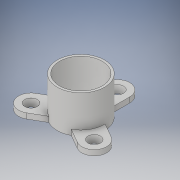
# Autodesk Inventor part: Wood Mount 1 Inch
Saved by Autodesk Inventor 2018 (Build 220112000, 112)
## iProperties
Created: 2018-01-10
Part Number: Wood Mount 1 Inch
Material: Generic
Document SubType Name: Modeling
Designer: owner
Density: 1 g/cm^3
Appearance: Default
Author: owner
Autodesk Inventor part; units mm, degrees
ref_plane "YZ Plane" through (0, 0, 0) normal (1, 0, 0) x (0, 1, 0)
ref_plane "XZ Plane" through (0, 0, 0) normal (0, 1, 0) x (-1, 0, 0)
sketch "Sketch1" plane through (0, 0, 0) normal (0, 1, 0) x (-1, 0, 0)
  circle A0 centre (0, 0) radius 16.7767
  circle A1 centre (0, 0) radius 18.5801
  circle A2 centre (-24.8666, 14.3567) radius 2.413
  circle A3 centre (-24.8666, 14.3567) radius 4.8895
  line L0 (-29.7371, 5.9209) -> (-18.5727, -0.5249)
  line L1 (-19.9962, 22.7926) -> (-8.8318, 16.3469)
  arc A4 (-19.9962, 22.7926) -> (-29.7371, 5.9209) centre (-24.8666, 14.3567) ccw
  circle A5 centre (0, -28.7135) radius 2.413
  circle A6 centre (0, -28.7135) radius 4.8895
  line L2 (-9.7409, -28.7135) -> (-9.7409, -15.822)
  arc A7 (-9.7409, -28.7135) -> (9.7409, -28.7135) centre (0, -28.7135) ccw
  line L3 (9.7409, -28.7135) -> (9.7409, -15.822)
  circle A8 centre (24.8666, 14.3567) radius 2.413
  circle A9 centre (24.8666, 14.3567) radius 4.8895
  line L4 (29.7371, 5.9209) -> (18.5727, -0.5249)
  arc A10 (29.7371, 5.9209) -> (19.9961, 22.7926) centre (24.8666, 14.3567) ccw
  line L5 (19.9961, 22.7926) -> (8.8318, 16.3469)
  point P0 (0, 14.3567)
  point P1 (-16.0908, 9.29)
  constraints: 12 end point, 10 centre point, 7 coincident, 6 point on circle, 1 tangent, 9 other
extrude "Extrusion1" add sketch "Sketch1" along normal blind 29.5402 contours A1
extrude "Extrusion2" add sketch "Sketch1" along normal blind 4.2164 contours A1 L0 A4 L1
extrude "Extrusion3" add sketch "Sketch1" along normal blind 4.2164 contours A1 L5 A10 L4
extrude "Extrusion4" add sketch "Sketch1" along normal blind 4.2164 contours L3 A7 L2 A1
sketch "Sketch2" plane through (0, 4.2164, 0) normal (0, 1, 0) x (1, 0, 0)
  arc A0 (-29.7371, -5.9209) -> (-19.9961, -22.7926) centre (-24.8666, -14.3567) ccw projected
  line L0 (-19.9961, -22.7926) -> (-8.8318, -16.3469) projected
  arc A1 (-18.5727, 0.5249) -> (-8.8318, -16.3469) centre (0, 0) ccw projected
  line L1 (-18.5727, 0.5249) -> (-29.7371, -5.9209) projected
  circle A2 centre (24.8666, -14.3567) radius 4.8895 projected
  circle A3 centre (0, 28.7135) radius 4.8895 projected
  arc A4 (9.7409, 28.7135) -> (-9.7409, 28.7135) centre (0, 28.7135) ccw projected
  line L2 (9.7409, 15.822) -> (9.7409, 28.7135) projected
  line L3 (-9.7409, 28.7135) -> (-9.7409, 15.822) projected
  circle A5 centre (0, 28.7135) radius 2.413 projected
  line L4 (29.7371, -5.9209) -> (18.5727, 0.5249) projected
  arc A6 (19.9962, -22.7926) -> (29.7371, -5.9209) centre (24.8666, -14.3567) ccw projected
  circle A7 centre (24.8666, -14.3567) radius 2.413 projected
  line L5 (8.8318, -16.3469) -> (19.9962, -22.7926) projected
  circle A8 centre (0, 0) radius 18.5801 projected
  circle A9 centre (0, 0) radius 16.7767 projected
ref_plane "Work Plane1" through (-13.7086, 0, 7.9) normal (0.5, 0, 0.866) x (0.866, 0, -0.5)
sketch "Sketch3" plane through (-13.7086, 0, 7.9) normal (0.5, 0, 0.866) x (0.866, 0, -0.5)
  line L0 (-10.4785, 0) -> (-15.3045, 0) projected
  line L1 (-10.4785, 0) -> (-8.002, 4.2164)
  line L2 (-8.002, 4.2164) -> (-8.002, 0)
  line L3 (-8.002, 0) -> (-8.002, 4.2164) projected
  line L4 (-8.002, 0) -> (-10.4785, 0)
  line L5 (-12.8915, 0) -> (-12.8915, 4.2164) projected
  line L6 (-12.8915, 0) -> (-12.8915, 8.5631)
  point P0 (15.822, 0)
  constraints: 8 end point, 2 collinear, 1 point on line
revolve "Revolution1" add sketch "Sketch3" angle 360 about axis through (-24.8729, 0, 14.3457) along (0, 1, 0)
ref_plane "Work Plane2" through (0, 0, 0) normal (0.5, 0, -0.866) x (0, 1, 0)
sketch "Sketch4" plane through (0, 0, 0) normal (0.5, 0, -0.866) x (0, 1, 0)
  line L0 (0, 26.3005) -> (0, 31.1265) projected
  line L1 (4.2164, 33.603) -> (4.2164, 23.824) projected
  line L2 (4.2164, 33.603) -> (0, 31.1265)
  line L3 (0, 23.824) -> (0, 33.603) projected
  line L4 (0, 31.1265) -> (0, 33.603)
  line L5 (0, 33.603) -> (4.2164, 33.603)
  line L6 (0, 28.7135) -> (10.3946, 28.7135)
  point P0 (0, 0)
  constraints: 8 end point, 1 horizontal, 1 midpoint, 1 perpendicular, 1 vertical
revolve "Revolution2" add sketch "Sketch4" angle 360 about axis through (24.8666, 0, 14.3567) along (0, 1, 0) contours L3 L5 L2
ref_plane "Work Plane3" through (0, 0, 0) normal (-1, 0, 0) x (0, 1, 0)
sketch "Sketch5" plane through (0, 0, 0) normal (-1, 0, 0) x (0, 1, 0)
  line L0 (0, 26.3005) -> (0, 31.1265) projected
  line L1 (4.2164, 33.603) -> (4.2164, 23.824) projected
  line L2 (0, 31.1265) -> (4.2164, 33.603)
  line L3 (0, 23.824) -> (0, 33.603) projected
  line L4 (4.2164, 33.603) -> (0, 33.603)
  line L5 (0, 33.603) -> (0, 31.1265)
  line L6 (0, 28.7135) -> (13.6215, 28.7135)
  point P0 (0, 0)
  constraints: 8 end point, 2 horizontal, 1 midpoint, 1 perpendicular
revolve "Revolution3" add sketch "Sketch5" angle 360 about axis through (0, 0, -28.7135) along (0, 1, 0) contours L3 L4 L2
body "Solid1"
